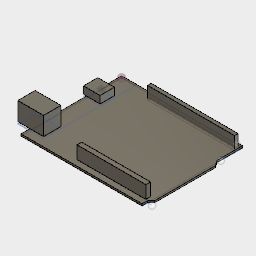
Arduino Model v1 (Autodesk Fusion 360 design; units mm, degrees)
Autodesk Fusion 360 part; units mm, degrees
sketch "Sketch1" plane through (0, 0, 0) normal (0, 1, 0) x (1, 0, 0)
  line L0 (0, 0) -> (66.09, 0)
  line L1 (66.09, 0) -> (66.09, -54.95)
  line L2 (66.09, -54.95) -> (0, -54.95)
  line L3 (0, -54.95) -> (0, 0)
  line L4 (66.09, 0) -> (65.09, 0)
  line L5 (65.09, 0) -> (65.09, -1.5)
  line L6 (65.09, -1.5) -> (66.09, -1.5)
  line L7 (66.09, -1.5) -> (66.09, 0)
  line L8 (65.09, -1.5) -> (17.59, -1.5)
  line L9 (17.59, -1.5) -> (17.59, -3.5)
  line L10 (17.59, -3.5) -> (65.09, -3.5)
  line L11 (65.09, -3.5) -> (65.09, -1.5)
  line L12 (0, 0) -> (7.5, 0)
  line L13 (0, -11) -> (0, 0)
  line L14 (66.09, 0) -> (62.5, 0)
  line L15 (66.09, 0) -> (66.09, -12)
  line L16 (66.09, -54.95) -> (66.09, -51.95)
  line L17 (66.09, -51.95) -> (68.59, -51.95)
  line L18 (7.5, 0) -> (7.5, -19.22)
  line L19 (7.5, -19.22) -> (-1.64, -19.22)
  line L20 (-1.64, -19.22) -> (-1.64, -11.37)
  line L21 (-1.64, -11.37) -> (7.5, -11.37)
  line L22 (7.5, -11.37) -> (7.5, -19.22)
  line L23 (7.5, -19.22) -> (7.5, -40.53)
  line L24 (7.5, -40.53) -> (-6.65, -40.53)
  line L25 (-6.65, -40.53) -> (-6.65, -50.06)
  line L26 (-6.65, -50.06) -> (7.5, -50.06)
  line L27 (7.5, -50.06) -> (7.5, -40.53)
  dimension "d1" = 54.95
  dimension "d2" = 66.09
  dimension "d3" = 1.5
  dimension "d4" = 1
  dimension "d5" = 47.5
  dimension "d6" = 2
  dimension "d7" = 11
  dimension "d8" = 7.5
  dimension "d21" = 12
  dimension "d24" = 3
  dimension "d25" = 2.5
  dimension "d27" = 19.22
  dimension "d28" = 7.85
  dimension "d29" = 9.14
  dimension "d30" = 21.31
  dimension "d31" = 14.15
  dimension "d32" = 9.53
  measures "d1" distance of L0.start L2.end
  measures "d2" distance of L0.start L0.end
  measures "d3" distance of L0.end L6.end
  measures "d4" distance of L0.end L4.end
  measures "d5" distance of L5.end L8.end
  measures "d6" distance of L5.end L10.end
  measures "d7" distance of L0.start L13.start
  measures "d8" distance of L0.start L12.end
  measures "d21" distance of L0.end L15.end
  measures "d24" distance of L1.end L16.end
  measures "d25" distance of L16.end L17.end
  measures "d27" distance of L12.end L18.end
  measures "d28" distance of L18.end L21.end
  measures "d29" distance of L18.end L19.end
  measures "d30" distance of L18.end L23.end
  measures "d31" distance of L23.end L24.end
  measures "d32" distance of L23.end L26.end
extrude "Extrude2" add sketch "Sketch1" along normal blind 7 contours L8 L9 L10 L11 makes body 1
extrude "Extrude1" add sketch "Sketch1" along normal blind 1 separate body contours L0 L3 L12 L13 L18 L21 | L8 L9 L10 L11 | L0 L1 L2 L3 L5 L6 L14 L15 L16 L18 L22 L23 L26 L27 | L3 L18 L19 L21 L22 | L0 L1 L4 L5 L6 L7 L14 L15 | L3 L19 L23 L24 | L3 L24 L26 L27 makes body 2
sketch "Sketch2" plane through (0, 1, 0) normal (0, 1, 0) x (-1, 0, 0)
  line L0 (-66.09, 54.95) -> (-66.09, 0)
  line L1 (-66.09, 0) -> (0, 0)
  line L2 (0, 0) -> (0, 54.95)
  line L3 (0, 54.95) -> (-66.09, 54.95)
  line L4 (-7.5, 50.06) -> (-7.5, 40.53)
  line L5 (6.65, 40.53) -> (-7.5, 40.53)
  line L6 (-7.5, 50.06) -> (6.65, 50.06)
  line L7 (6.65, 50.06) -> (6.65, 40.53)
  point P0 (6.65, 40.53)
  point P1 (-7.5, 40.53)
  point P2 (6.65, 50.06)
extrude "Extrude4" add sketch "Sketch2" along normal blind 10 contours L2 L5 L6 L7 | L2 L4 L5 L6 bodies 2
sketch "Sketch3" plane through (0, 1, 0) normal (0, 1, 0) x (-1, 0, 0)
  line L0 (-7.5, 50.06) -> (0, 50.06)
  line L1 (0, 50.06) -> (0, 54.95)
  line L2 (0, 54.95) -> (-66.09, 54.95)
  line L3 (-66.09, 54.95) -> (-66.09, 0)
  line L4 (-66.09, 0) -> (0, 0)
  line L5 (0, 0) -> (0, 40.53)
  line L6 (0, 40.53) -> (-7.5, 40.53)
  line L7 (-7.5, 40.53) -> (-7.5, 50.06)
  line L8 (1.64, 11.37) -> (-7.5, 11.37)
  line L9 (-7.5, 11.37) -> (-7.5, 19.22)
  line L10 (-7.5, 19.22) -> (1.64, 19.22)
  line L11 (1.64, 19.22) -> (1.64, 11.37)
  point P0 (1.64, 11.37)
  point P1 (-7.5, 19.22)
extrude "Extrude5" add sketch "Sketch3" along normal blind 4 contours L5 L8 L10 L11 | L5 L8 L9 L10 bodies 2
sketch "Sketch4" plane through (0, 1, 0) normal (0, 1, 0) x (-1, 0, 0)
  line L0 (-7.5, 19.22) -> (0, 19.22)
  line L1 (0, 19.22) -> (0, 40.53)
  line L2 (0, 40.53) -> (-7.5, 40.53)
  line L3 (-7.5, 40.53) -> (-7.5, 50.06)
  line L4 (-7.5, 50.06) -> (0, 50.06)
  line L5 (0, 50.06) -> (0, 54.95)
  line L6 (0, 54.95) -> (-66.09, 54.95)
  line L7 (-66.09, 54.95) -> (-66.09, 0)
  line L8 (-66.09, 0) -> (0, 0)
  line L9 (0, 0) -> (0, 11.37)
  line L10 (0, 11.37) -> (-7.5, 11.37)
  line L11 (-7.5, 11.37) -> (-7.5, 19.22)
  line L12 (-65.09, 3.5) -> (-65.09, 49.3)
  line L13 (-65.09, 49.3) -> (-27.52, 49.3)
  line L14 (-27.52, 49.3) -> (-27.52, 51.83)
  line L15 (-27.52, 51.83) -> (-65.09, 51.83)
  line L16 (-65.09, 51.83) -> (-65.09, 49.3)
  point P0 (-65.09, 3.5)
  dimension "d37" = 45.8
  dimension "d38" = 37.57
  dimension "d39" = 2.53
  measures "d37" distance of P0 L12.end
  measures "d38" distance of L12.end L13.end
  measures "d39" distance of L12.end L15.end
extrude "Extrude6" add sketch "Sketch4" along normal blind 7 contours L13 L14 L15 L16 bodies 2
sketch "Sketch5" plane through (0, 1, 0) normal (0, 1, 0) x (-1, 0, 0)
  line L0 (-65.09, 51.83) -> (-27.52, 51.83)
  line L1 (-27.52, 51.83) -> (-27.52, 49.3)
  line L2 (-27.52, 49.3) -> (-65.09, 49.3)
  line L3 (-65.09, 49.3) -> (-65.09, 51.83)
  line L4 (-7.5, 19.22) -> (0, 19.22)
  line L5 (0, 19.22) -> (0, 40.53)
  line L6 (0, 40.53) -> (-7.5, 40.53)
  line L7 (-7.5, 40.53) -> (-7.5, 50.06)
  line L8 (-7.5, 50.06) -> (0, 50.06)
  line L9 (0, 50.06) -> (0, 54.95)
  line L10 (0, 54.95) -> (-66.09, 54.95)
  line L11 (-66.09, 54.95) -> (-66.09, 0)
  line L12 (-66.09, 0) -> (0, 0)
  line L13 (0, 0) -> (0, 11.37)
  line L14 (0, 11.37) -> (-7.5, 11.37)
  line L15 (-7.5, 11.37) -> (-7.5, 19.22)
  line L16 (-66.09, 54.95) -> (-66.09, 51.95)
  line L17 (-66.09, 51.95) -> (-68.09, 49.95)
  line L18 (-68.09, 49.95) -> (-68.09, 16.95)
  line L19 (-68.09, 16.95) -> (-66.09, 16.95)
  line L20 (-66.09, 0) -> (-68.09, 0)
  line L21 (-66.09, 0) -> (-66.09, 14)
  line L22 (-66.09, 14) -> (-68.09, 16.95)
  dimension "d44" = 3
  dimension "d45" = 33
  dimension "d46" = 14
  measures "d44" distance of L10.end L16.end
  measures "d45" distance of L17.end L18.end
  measures "d46" distance of L11.end L21.end
extrude "Extrude7" add sketch "Sketch5" against normal blind 1 contours L11 L19 L22 | L11 L17 L18 L19 bodies 2
